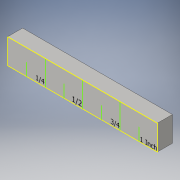
# Autodesk Inventor part: 1 inch Ruler
Saved by Autodesk Inventor 2016 (Build 200138000, 138)
## iProperties
Created: 2015-07-25
Part Number: 1 inch Ruler
Material: Generic
Document SubType Name: Modeling
Designer: Nancy
Density: 1 g/cm^3
Appearance: Default
Author: Nancy
Autodesk Inventor part; units mm, degrees
ref_plane "YZ Plane" through (0, 0, 0) normal (1, 0, 0) x (0, 1, 0)
ref_plane "XZ Plane" through (0, 0, 0) normal (0, 1, 0) x (-1, 0, 0)
ref_plane "XY Plane" through (0, 0, 0) normal (0, 0, 1) x (1, 0, 0)
sketch "Sketch1" plane through (0, 0, 0) normal (0, 0, 1) x (1, 0, 0)
  line L0 (0, 0) -> (25.4, 0)
  line L1 (25.4, 0) -> (25.4, 4.2333)
  line L2 (25.4, 4.2333) -> (0, 4.2333)
  line L3 (0, 4.2333) -> (0, 0)
  dimension "d0" = 25.4
  dimension "d1" = 4.2333
  constraints: 8 end point, 2 parallel, 1 horizontal, 1 perpendicular
  measures "d0" distance of L0.start L0.end
  measures "d1" distance of L2.end L0.start
extrude "Extrusion1" add sketch "Sketch1" along normal blind 2.54
sketch "Sketch2" plane through (0, 0, 2.54) normal (0, 0, 1) x (1, 0, 0)
  line L0 (0, 0) -> (25.4, 0) projected
  line L1 (12.7, 0) -> (12.7, 4.2333)
  line L2 (25.4, 4.2333) -> (0, 4.2333) projected
  line L3 (25.4, 0) -> (25.4, 4.2333) projected
  line L4 (6.35, 0) -> (6.35, 4.2333)
  line L5 (19.05, 0) -> (19.05, 4.2333)
  line L6 (0, 4.2333) -> (0, 0) projected
  line L7 (10.8658, 1.0986) -> (12.7, 1.0986) construction
  line L8 (12.7, 1.0986) -> (12.7, 0) construction
  line L9 (12.7, 0) -> (10.8658, 0) construction
  line L10 (10.8658, 0) -> (10.8658, 1.0986) construction
  line L11 (4.7138, 1.0986) -> (6.2582, 1.0986) construction
  line L12 (6.2582, 1.0986) -> (6.2582, 0.1371) construction
  line L13 (6.2582, 0.1371) -> (4.7138, 0.1371) construction
  line L14 (4.7138, 0.1371) -> (4.7138, 1.0986) construction
  line L15 (17.4571, 1.0187) -> (19.0015, 1.0187) construction
  line L16 (19.0015, 1.0187) -> (19.0015, 0.0572) construction
  line L17 (19.0015, 0.0572) -> (17.4571, 0.0572) construction
  line L18 (17.4571, 0.0572) -> (17.4571, 1.0187) construction
  line L19 (3.175, 0) -> (3.175, 2.1167)
  line L20 (9.525, 0) -> (9.525, 2.1167)
  line L21 (15.875, 0) -> (15.875, 2.1082)
  line L22 (22.225, 0) -> (22.225, 2.1082)
  line L23 (22.4144, 0.8901) -> (25.3778, 0.8901) construction
  line L24 (25.3778, 0.8901) -> (25.3778, 0.007) construction
  line L25 (25.3778, 0.007) -> (22.4144, 0.007) construction
  line L26 (22.4144, 0.007) -> (22.4144, 0.8901) construction
  constraints: 14 end point, 5 vertical, 2 perpendicular, 2 point on line, 1 coincident, 1 midpoint, 16 other
body "Solid1"
